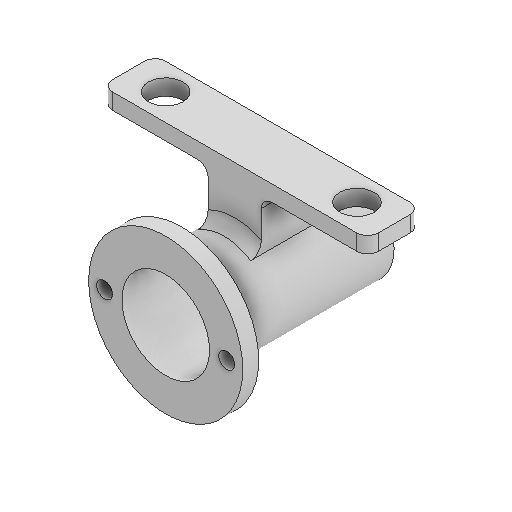
# Autodesk Inventor part: AcopleTC
Saved by Autodesk Inventor 2025.2 (Build 292293000, 293)
## iProperties
Created: 2025-11-03
Part Number: AcopleTC
Material: Generic
Document SubType Name: Modeling
Designer: Compa
Density: 1 g/cm^3
Appearance: Default
Author: Compa
Autodesk Inventor part; units mm, degrees
ref_plane "YZ Plane" through (0, 0, 0) normal (1, 0, 0) x (0, 1, 0)
ref_plane "XY Plane" through (0, 0, 0) normal (0, 0, 1) x (1, 0, 0)
sketch "Sketch1" plane through (0, 0, 0) normal (0, 0, 1) x (1, 0, 0)
  circle A0 centre (0, 0) radius 14.5
  circle A1 centre (11.5, 0) radius 1.5
  line L0 (0, 16.0858) -> (0, -16.9174) construction
  line L1 (-27.4443, 0) -> (33.7473, 0) construction
  circle A2 centre (-11.5, 0) radius 1.5
  circle A3 centre (0, 0) radius 8.25
  dimension "d0" = 29
  dimension "d1" = 3
  dimension "d2" = 11.5
  dimension "d3" = 16.5
  constraints: 4 centre point, 4 end point, 2 coincident, 2 horizontal, 2 vertical, 1 symmetric about line, 1 other
  measures "d0" diameter of A0
  measures "d1" diameter of A1
  measures "d2" distance of A1.centre point (0, 0)
  measures "d3" diameter of A3
extrude "Extrusion1" add sketch "Sketch1" along normal blind 3
sketch "Sketch2" plane through (0, 0, 0) normal (0, 0, -1) x (-1, 0, 0)
  circle A0 centre (0, 0) radius 9
  dimension "d6" = 18
  constraints: 1 centre point, 1 coincident
  measures "d6" diameter of A0
extrude "Extrusion2" add sketch "Sketch2" along normal blind 31
fillet "Fillet1" radius 2 1 edges at (9, 0, 0)
sketch "Sketch3" plane through (0, 0, 0) normal (0, 0, 1) x (1, 0, 0)
  circle A0 centre (0, 0) radius 8.25 projected
extrude "Extrusion3" cut sketch "Sketch3" against normal blind 30
ref_plane "Work Plane1" through (0, 20, 0) normal (0, 1, 0) x (-1, 0, 0)
sketch "Sketch5" plane through (0, 20, 0) normal (0, 1, 0) x (-1, 0, 0)
  line L0 (-25, -10) -> (25, -10)
  line L1 (25, -10) -> (25, -20)
  line L2 (25, -20) -> (-25, -20)
  line L3 (-25, -20) -> (-25, -10)
  line L4 (-25, -10) -> (25, -20) construction
  line L5 (25, -10) -> (-25, -20) construction
  point P0 (0, 0)
  point P1 (0, -15)
  dimension "d19" = 50
  dimension "d20" = 10
  dimension "d27" = 15
  constraints: 12 end point, 2 midpoint, 2 parallel, 1 horizontal, 1 perpendicular
  measures "d19" distance of L1.end L2.end
  measures "d20" distance of L0.end L1.end
  measures "d27" distance of point (0, 0) point (0, -15)
extrude "Extrusion5" add sketch "Sketch5" against normal blind 3
fillet "Fillet3" radius 2 4 edges at (-25, 18.5, -10) (-25, 18.5, -20) (25, 18.5, -10) (25, 18.5, -20)
sketch "Sketch6" plane through (0, 17, 0) normal (0, -1, 0) x (1, 0, 0)
  line L0 (-5, -20) -> (5, -20)
  line L1 (5, -20) -> (5, -10)
  line L2 (5, -10) -> (-5, -10)
  line L3 (-5, -10) -> (-5, -20)
  line L4 (-5, -20) -> (5, -10) construction
  line L5 (5, -20) -> (-5, -10) construction
  point P0 (0, 0)
  point P1 (0, -15)
  dimension "d24" = 10
  dimension "d25" = 10
  dimension "d26" = 15
  constraints: 12 end point, 2 midpoint, 2 parallel, 1 horizontal, 1 perpendicular
  measures "d24" distance of L2.end L1.end
  measures "d25" distance of L1.end L0.end
  measures "d26" distance of point (0, 0) point (0, -15)
extrude "Extrusion6" add sketch "Sketch6" along normal up to next
fillet "Fillet4" radius 2 2 edges at (5, 17, -15) (-5, 17, -15)
fillet "Fillet5" radius 2 2 edges at (0, 9, -10) (0, 9, -20)
sketch "Sketch7" plane through (0, 20, 0) normal (0, 1, 0) x (1, 0, 0)
  circle A0 centre (18, 15) radius 3.25
  circle A1 centre (-18, 15) radius 3.25
  line L0 (0, -10.182) -> (0, 25.8871) construction
  line L1 (-23, 10) -> (23, 10) projected
  point P0 (0, 0)
  dimension "d32" = 6.5
  dimension "d33" = 6.5
  dimension "d34" = 36
  dimension "d35" = 5
  constraints: 2 centre point, 2 end point, 2 vertical, 1 symmetric about line
  measures "d32" diameter of A0
  measures "d33" diameter of A1
  measures "d34" distance of A1.centre A0.centre
  measures "d35" distance from line of L1 A0.centre
extrude "Extrusion7" cut sketch "Sketch7" against normal blind 10
body "Solid1"
